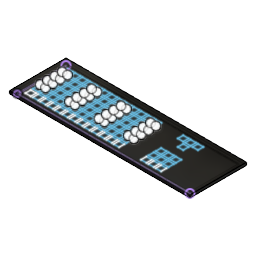
keyboard (Autodesk Fusion 360 design; units mm, degrees)
part number: 2026-07-05-21-32-07-139
Autodesk Fusion 360 part; units mm, degrees
sketch "Sketch1" plane through (0, 0, 0) normal (0, 1, 0) x (1, 0, 0)
  line L0 (0, 0) -> (446, 0)
  line L1 (446, 0) -> (446, -126)
  line L2 (446, -126) -> (0, -126)
  line L3 (0, -126) -> (0, 0)
  line L4 (-10, 10) -> (456, 10)
  line L5 (456, 10) -> (456, -136)
  line L6 (456, -136) -> (-10, -136)
  line L7 (-10, -136) -> (-10, 10)
  dimension "d1" = 446
  dimension "d2" = 126
  dimension "d3" = 466
  dimension "d4" = 146
  dimension "d5" = 10
  dimension "d6" = 10
  constraint horizontal L0
  constraint vertical L1
  constraint horizontal L2
  constraint vertical L3
  constraint coincident L0.start L3.end
  constraint horizontal L4
  constraint vertical L5
  constraint horizontal L6
  constraint vertical L7
  measures "d1" distance of L0.start L0.end
  measures "d2" distance of L0.start L2.end
  measures "d3" distance of L4.start L4.end
  measures "d4" distance of L4.start L6.end
  measures "d5" distance of L3 L7
  measures "d6" distance of L0 L4
extrude "Extrude1" add sketch "Sketch1" along normal blind 5 contours L0 L1 L2 L3 | L4 L5 L6 L7
extrude "Extrude2" cut sketch "Sketch1" along normal blind 4 contours L0 L1 L2 L3
extrude "Extrude3" add 1 faces at (145.3333, 5, 38.6667) along direction (0, 1, 0) blind 2
sketch "Sketch2" plane through (0, 0, 0) normal (0, 1, 0) x (1, 0, 0)
  line L0 (9, -114) -> (23, -114)
  line L1 (23, -114) -> (23, -100)
  line L2 (23, -100) -> (9, -100)
  line L3 (9, -100) -> (9, -114)
  line L4 (28, -113.6288) -> (42, -113.6288)
  line L5 (42, -113.6288) -> (42, -99.6288)
  line L6 (42, -99.6288) -> (28, -99.6288)
  line L7 (28, -99.6288) -> (28, -113.6288)
  line L8 (0, 0) -> (0, -126)
  line L9 (0, -126) -> (446, -126)
  line L10 (47, -113.6288) -> (61, -113.6288)
  line L11 (47, -99.6288) -> (47, -113.6288)
  line L12 (61, -113.6288) -> (61, -99.6288)
  line L13 (61, -99.6288) -> (47, -99.6288)
  line L14 (80, -113.6288) -> (80, -99.6288)
  line L15 (66, -113.6288) -> (80, -113.6288)
  line L16 (66, -99.6288) -> (66, -113.6288)
  line L17 (80, -99.6288) -> (66, -99.6288)
  line L18 (156, -113.6288) -> (156, -99.6288)
  line L19 (142, -113.6288) -> (156, -113.6288)
  line L20 (142, -99.6288) -> (142, -113.6288)
  line L21 (156, -99.6288) -> (142, -99.6288)
  line L22 (137, -113.6288) -> (137, -99.6288)
  line L23 (123, -99.6288) -> (123, -113.6288)
  line L24 (123, -113.6288) -> (137, -113.6288)
  line L25 (137, -99.6288) -> (123, -99.6288)
  line L26 (118, -113.6288) -> (118, -99.6288)
  line L27 (104, -113.6288) -> (118, -113.6288)
  line L28 (104, -99.6288) -> (104, -113.6288)
  line L29 (118, -99.6288) -> (104, -99.6288)
  line L30 (99, -114) -> (99, -100)
  line L31 (85, -114) -> (99, -114)
  line L32 (85, -100) -> (85, -114)
  line L33 (99, -100) -> (85, -100)
  line L34 (307.2, -113.6288) -> (321.2, -113.6288)
  line L35 (218, -113.6288) -> (232, -113.6288)
  line L36 (345.2, -113.6288) -> (359.2, -113.6288)
  line L37 (307.2, -99.6288) -> (307.2, -113.6288)
  line L38 (161, -114) -> (175, -114)
  line L39 (232, -113.6288) -> (232, -99.6288)
  line L40 (345.2, -99.6288) -> (345.2, -113.6288)
  line L41 (359.2, -99.6288) -> (345.2, -99.6288)
  line L42 (340.2, -113.6288) -> (340.2, -99.6288)
  line L43 (326.2, -99.6288) -> (326.2, -113.6288)
  line L44 (326.2, -113.6288) -> (340.2, -113.6288)
  line L45 (359.2, -113.6288) -> (359.2, -99.6288)
  line L46 (340.2, -99.6288) -> (326.2, -99.6288)
  line L47 (321.2, -113.6288) -> (321.2, -99.6288)
  line L48 (237, -114) -> (251, -114)
  line L49 (251, -114) -> (251, -100)
  line L50 (321.2, -99.6288) -> (307.2, -99.6288)
  line L51 (232, -99.6288) -> (218, -99.6288)
  line L52 (237, -100) -> (237, -114)
  line L53 (251, -100) -> (237, -100)
  line L54 (161, -100) -> (161, -114)
  line L55 (175, -114) -> (175, -100)
  line L56 (175, -100) -> (161, -100)
  line L57 (180, -99.6288) -> (180, -113.6288)
  line L58 (218, -99.6288) -> (218, -113.6288)
  line L59 (194, -113.6288) -> (194, -99.6288)
  line L60 (199, -113.6288) -> (213, -113.6288)
  line L61 (199, -99.6288) -> (199, -113.6288)
  line L62 (213, -113.6288) -> (213, -99.6288)
  line L63 (213, -99.6288) -> (199, -99.6288)
  line L64 (180, -113.6288) -> (194, -113.6288)
  line L65 (194, -99.6288) -> (180, -99.6288)
  line L66 (321.2, -94.6288) -> (321.2, -80.6288)
  line L67 (85, -95) -> (99, -95)
  line L68 (307.2, -80.6288) -> (307.2, -94.6288)
  line L69 (345.2, -94.6288) -> (359.2, -94.6288)
  line L70 (85, -81) -> (85, -95)
  line L71 (80, -80.6288) -> (66, -80.6288)
  line L72 (326.2, -94.6288) -> (340.2, -94.6288)
  line L73 (66, -94.6288) -> (80, -94.6288)
  line L74 (321.2, -80.6288) -> (307.2, -80.6288)
  line L75 (251, -95) -> (251, -81)
  line L76 (307.2, -94.6288) -> (321.2, -94.6288)
  line L77 (175, -81) -> (161, -81)
  line L78 (345.2, -80.6288) -> (345.2, -94.6288)
  line L79 (237, -81) -> (237, -95)
  line L80 (340.2, -94.6288) -> (340.2, -80.6288)
  line L81 (326.2, -80.6288) -> (326.2, -94.6288)
  line L82 (194, -80.6288) -> (180, -80.6288)
  line L83 (175, -95) -> (175, -81)
  line L84 (199, -80.6288) -> (199, -94.6288)
  line L85 (218, -94.6288) -> (232, -94.6288)
  line L86 (359.2, -80.6288) -> (345.2, -80.6288)
  line L87 (180, -80.6288) -> (180, -94.6288)
  line L88 (194, -94.6288) -> (194, -80.6288)
  line L89 (237, -95) -> (251, -95)
  line L90 (232, -94.6288) -> (232, -80.6288)
  line L91 (218, -80.6288) -> (218, -94.6288)
  line L92 (340.2, -80.6288) -> (326.2, -80.6288)
  line L93 (213, -80.6288) -> (199, -80.6288)
  line L94 (161, -95) -> (175, -95)
  line L95 (251, -81) -> (237, -81)
  line L96 (156, -94.6288) -> (156, -80.6288)
  line L97 (199, -94.6288) -> (213, -94.6288)
  line L98 (213, -94.6288) -> (213, -80.6288)
  line L99 (232, -80.6288) -> (218, -80.6288)
  line L100 (161, -81) -> (161, -95)
  line L101 (180, -94.6288) -> (194, -94.6288)
  line L102 (61, -94.6288) -> (61, -80.6288)
  line L103 (156, -80.6288) -> (142, -80.6288)
  line L104 (42, -80.6288) -> (28, -80.6288)
  line L105 (28, -80.6288) -> (28, -94.6288)
  line L106 (9, -81) -> (9, -95)
  line L107 (142, -94.6288) -> (156, -94.6288)
  line L108 (61, -80.6288) -> (47, -80.6288)
  line L109 (23, -81) -> (9, -81)
  line L110 (47, -94.6288) -> (61, -94.6288)
  line L111 (66, -80.6288) -> (66, -94.6288)
  line L112 (47, -80.6288) -> (47, -94.6288)
  line L113 (9, -95) -> (23, -95)
  line L114 (123, -80.6288) -> (123, -94.6288)
  line L115 (42, -94.6288) -> (42, -80.6288)
  line L116 (28, -94.6288) -> (42, -94.6288)
  line L117 (23, -95) -> (23, -81)
  line L118 (118, -94.6288) -> (118, -80.6288)
  line L119 (137, -80.6288) -> (123, -80.6288)
  line L120 (99, -81) -> (85, -81)
  line L121 (123, -94.6288) -> (137, -94.6288)
  line L122 (104, -94.6288) -> (118, -94.6288)
  line L123 (104, -80.6288) -> (104, -94.6288)
  line L124 (137, -94.6288) -> (137, -80.6288)
  line L125 (80, -94.6288) -> (80, -80.6288)
  line L126 (142, -80.6288) -> (142, -94.6288)
  line L127 (118, -80.6288) -> (104, -80.6288)
  line L128 (359.2, -94.6288) -> (359.2, -80.6288)
  line L129 (99, -95) -> (99, -81)
  line L130 (237, -62) -> (237, -76)
  line L131 (232, -61.6288) -> (218, -61.6288)
  line L132 (251, -62) -> (237, -62)
  line L133 (213, -75.6288) -> (213, -61.6288)
  line L134 (194, -75.6288) -> (194, -61.6288)
  line L135 (180, -61.6288) -> (180, -75.6288)
  line L136 (175, -62) -> (161, -62)
  line L137 (156, -75.6288) -> (156, -61.6288)
  line L138 (194, -61.6288) -> (180, -61.6288)
  line L139 (161, -62) -> (161, -76)
  line L140 (251, -76) -> (251, -62)
  line L141 (218, -61.6288) -> (218, -75.6288)
  line L142 (232, -75.6288) -> (232, -61.6288)
  line L143 (218, -75.6288) -> (232, -75.6288)
  line L144 (326.2, -61.6288) -> (326.2, -75.6288)
  line L145 (307.2, -61.6288) -> (307.2, -75.6288)
  line L146 (359.2, -75.6288) -> (359.2, -61.6288)
  line L147 (359.2, -61.6288) -> (345.2, -61.6288)
  line L148 (156, -61.6288) -> (142, -61.6288)
  line L149 (142, -75.6288) -> (156, -75.6288)
  line L150 (307.2, -75.6288) -> (321.2, -75.6288)
  line L151 (326.2, -75.6288) -> (340.2, -75.6288)
  line L152 (340.2, -61.6288) -> (326.2, -61.6288)
  line L153 (321.2, -61.6288) -> (307.2, -61.6288)
  line L154 (199, -75.6288) -> (213, -75.6288)
  line L155 (213, -61.6288) -> (199, -61.6288)
  line L156 (104, -75.6288) -> (118, -75.6288)
  line L157 (118, -75.6288) -> (118, -61.6288)
  line L158 (345.2, -75.6288) -> (359.2, -75.6288)
  line L159 (137, -75.6288) -> (137, -61.6288)
  line L160 (42, -75.6288) -> (42, -61.6288)
  line L161 (99, -76) -> (99, -62)
  line L162 (99, -62) -> (85, -62)
  line L163 (66, -61.6288) -> (66, -75.6288)
  line L164 (123, -61.6288) -> (123, -75.6288)
  line L165 (47, -75.6288) -> (61, -75.6288)
  line L166 (80, -75.6288) -> (80, -61.6288)
  line L167 (142, -61.6288) -> (142, -75.6288)
  line L168 (66, -75.6288) -> (80, -75.6288)
  line L169 (42, -61.6288) -> (28, -61.6288)
  line L170 (345.2, -61.6288) -> (345.2, -75.6288)
  line L171 (340.2, -75.6288) -> (340.2, -61.6288)
  line L172 (321.2, -75.6288) -> (321.2, -61.6288)
  line L173 (123, -75.6288) -> (137, -75.6288)
  line L174 (118, -61.6288) -> (104, -61.6288)
  line L175 (137, -61.6288) -> (123, -61.6288)
  line L176 (104, -61.6288) -> (104, -75.6288)
  line L177 (85, -62) -> (85, -76)
  line L178 (80, -61.6288) -> (66, -61.6288)
  line L179 (28, -75.6288) -> (42, -75.6288)
  line L180 (9, -62) -> (9, -76)
  line L181 (23, -62) -> (9, -62)
  line L182 (47, -61.6288) -> (47, -75.6288)
  line L183 (23, -76) -> (23, -62)
  line L184 (61, -61.6288) -> (47, -61.6288)
  line L185 (28, -61.6288) -> (28, -75.6288)
  line L186 (61, -75.6288) -> (61, -61.6288)
  line L187 (199, -61.6288) -> (199, -75.6288)
  line L188 (175, -76) -> (175, -62)
  line L189 (180, -75.6288) -> (194, -75.6288)
  line L190 (9, -76) -> (23, -76)
  line L191 (85, -76) -> (99, -76)
  line L192 (161, -76) -> (175, -76)
  line L193 (237, -76) -> (251, -76)
  line L194 (213, -42.6288) -> (199, -42.6288)
  line L195 (66, -56.6288) -> (80, -56.6288)
  line L196 (104, -56.6288) -> (118, -56.6288)
  line L197 (251, -43) -> (237, -43)
  line L198 (9, -43) -> (9, -57)
  line L199 (47, -42.6288) -> (47, -56.6288)
  line L200 (213, -56.6288) -> (213, -42.6288)
  line L201 (42, -42.6288) -> (28, -42.6288)
  line L202 (28, -42.6288) -> (28, -56.6288)
  line L203 (61, -56.6288) -> (61, -42.6288)
  line L204 (232, -56.6288) -> (232, -42.6288)
  line L205 (232, -42.6288) -> (218, -42.6288)
  line L206 (28, -56.6288) -> (42, -56.6288)
  line L207 (180, -42.6288) -> (180, -56.6288)
  line L208 (80, -42.6288) -> (66, -42.6288)
  line L209 (237, -43) -> (237, -57)
  line L210 (47, -56.6288) -> (61, -56.6288)
  line L211 (237, -57) -> (251, -57)
  line L212 (218, -42.6288) -> (218, -56.6288)
  line L213 (118, -42.6288) -> (104, -42.6288)
  line L214 (199, -56.6288) -> (213, -56.6288)
  line L215 (218, -56.6288) -> (232, -56.6288)
  line L216 (23, -57) -> (23, -43)
  line L217 (61, -42.6288) -> (47, -42.6288)
  line L218 (251, -57) -> (251, -43)
  line L219 (23, -43) -> (9, -43)
  line L220 (42, -56.6288) -> (42, -42.6288)
  line L221 (9, -57) -> (23, -57)
  line L222 (66, -42.6288) -> (66, -56.6288)
  line L223 (104, -42.6288) -> (104, -56.6288)
  line L224 (142, -56.6288) -> (156, -56.6288)
  line L225 (156, -42.6288) -> (142, -42.6288)
  line L226 (85, -57) -> (99, -57)
  line L227 (85, -43) -> (85, -57)
  line L228 (194, -56.6288) -> (194, -42.6288)
  line L229 (99, -57) -> (99, -43)
  line L230 (199, -42.6288) -> (199, -56.6288)
  line L231 (194, -42.6288) -> (180, -42.6288)
  line L232 (175, -43) -> (161, -43)
  line L233 (161, -43) -> (161, -57)
  line L234 (80, -56.6288) -> (80, -42.6288)
  line L235 (99, -43) -> (85, -43)
  line L236 (180, -56.6288) -> (194, -56.6288)
  line L237 (156, -56.6288) -> (156, -42.6288)
  line L238 (175, -57) -> (175, -43)
  line L239 (137, -56.6288) -> (137, -42.6288)
  line L240 (123, -56.6288) -> (137, -56.6288)
  line L241 (118, -56.6288) -> (118, -42.6288)
  line L242 (123, -42.6288) -> (123, -56.6288)
  line L243 (142, -42.6288) -> (142, -56.6288)
  line L244 (161, -57) -> (175, -57)
  line L245 (137, -42.6288) -> (123, -42.6288)
  line L246 (237, -5) -> (237, -19)
  line L247 (237, -38) -> (251, -38)
  line L248 (218, -37.6288) -> (232, -37.6288)
  line L249 (199, -37.6288) -> (213, -37.6288)
  line L250 (237, -24) -> (237, -38)
  line L251 (156, -4.6288) -> (142, -4.6288)
  line L252 (23, -19) -> (23, -5)
  line L253 (218, -18.6288) -> (232, -18.6288)
  line L254 (251, -24) -> (237, -24)
  line L255 (47, -4.6288) -> (47, -18.6288)
  line L256 (251, -5) -> (237, -5)
  line L257 (142, -18.6288) -> (156, -18.6288)
  line L258 (213, -37.6288) -> (213, -23.6288)
  line L259 (232, -23.6288) -> (218, -23.6288)
  line L260 (213, -18.6288) -> (213, -4.6288)
  line L261 (218, -4.6288) -> (218, -18.6288)
  line L262 (251, -19) -> (251, -5)
  line L263 (237, -19) -> (251, -19)
  line L264 (156, -23.6288) -> (142, -23.6288)
  line L265 (251, -38) -> (251, -24)
  line L266 (213, -4.6288) -> (199, -4.6288)
  line L267 (232, -4.6288) -> (218, -4.6288)
  line L268 (232, -18.6288) -> (232, -4.6288)
  line L269 (232, -37.6288) -> (232, -23.6288)
  line L270 (218, -23.6288) -> (218, -37.6288)
  line L271 (199, -18.6288) -> (213, -18.6288)
  line L272 (213, -23.6288) -> (199, -23.6288)
  line L273 (61, -18.6288) -> (61, -4.6288)
  line L274 (42, -18.6288) -> (42, -4.6288)
  line L275 (137, -18.6288) -> (137, -4.6288)
  line L276 (9, -5) -> (9, -19)
  line L277 (28, -4.6288) -> (28, -18.6288)
  line L278 (61, -4.6288) -> (47, -4.6288)
  line L279 (137, -4.6288) -> (123, -4.6288)
  line L280 (118, -18.6288) -> (118, -4.6288)
  line L281 (99, -19) -> (99, -5)
  line L282 (66, -37.6288) -> (80, -37.6288)
  line L283 (80, -23.6288) -> (66, -23.6288)
  line L284 (66, -18.6288) -> (80, -18.6288)
  line L285 (28, -18.6288) -> (42, -18.6288)
  line L286 (118, -23.6288) -> (104, -23.6288)
  line L287 (9, -19) -> (23, -19)
  line L288 (9, -24) -> (9, -38)
  line L289 (142, -4.6288) -> (142, -18.6288)
  line L290 (104, -4.6288) -> (104, -18.6288)
  line L291 (66, -4.6288) -> (66, -18.6288)
  line L292 (47, -23.6288) -> (47, -37.6288)
  line L293 (80, -18.6288) -> (80, -4.6288)
  line L294 (80, -4.6288) -> (66, -4.6288)
  line L295 (85, -5) -> (85, -19)
  line L296 (99, -5) -> (85, -5)
  line L297 (123, -4.6288) -> (123, -18.6288)
  line L298 (118, -4.6288) -> (104, -4.6288)
  line L299 (23, -5) -> (9, -5)
  line L300 (42, -4.6288) -> (28, -4.6288)
  line L301 (175, -38) -> (175, -24)
  line L302 (142, -37.6288) -> (156, -37.6288)
  line L303 (175, -24) -> (161, -24)
  line L304 (156, -37.6288) -> (156, -23.6288)
  line L305 (180, -23.6288) -> (180, -37.6288)
  line L306 (161, -19) -> (175, -19)
  line L307 (180, -18.6288) -> (194, -18.6288)
  line L308 (175, -5) -> (161, -5)
  line L309 (194, -4.6288) -> (180, -4.6288)
  line L310 (175, -19) -> (175, -5)
  line L311 (161, -24) -> (161, -38)
  line L312 (194, -37.6288) -> (194, -23.6288)
  line L313 (194, -23.6288) -> (180, -23.6288)
  line L314 (199, -23.6288) -> (199, -37.6288)
  line L315 (194, -18.6288) -> (194, -4.6288)
  line L316 (161, -5) -> (161, -19)
  line L317 (180, -4.6288) -> (180, -18.6288)
  line L318 (199, -4.6288) -> (199, -18.6288)
  line L319 (156, -18.6288) -> (156, -4.6288)
  line L320 (180, -37.6288) -> (194, -37.6288)
  line L321 (161, -38) -> (175, -38)
  line L322 (66, -23.6288) -> (66, -37.6288)
  line L323 (104, -23.6288) -> (104, -37.6288)
  line L324 (9, -38) -> (23, -38)
  line L325 (137, -23.6288) -> (123, -23.6288)
  line L326 (23, -38) -> (23, -24)
  line L327 (85, -24) -> (85, -38)
  line L328 (42, -37.6288) -> (42, -23.6288)
  line L329 (23, -24) -> (9, -24)
  line L330 (104, -37.6288) -> (118, -37.6288)
  line L331 (118, -37.6288) -> (118, -23.6288)
  line L332 (47, -18.6288) -> (61, -18.6288)
  line L333 (123, -18.6288) -> (137, -18.6288)
  line L334 (28, -23.6288) -> (28, -37.6288)
  line L335 (142, -23.6288) -> (142, -37.6288)
  line L336 (104, -18.6288) -> (118, -18.6288)
  line L337 (123, -23.6288) -> (123, -37.6288)
  line L338 (99, -38) -> (99, -24)
  line L339 (123, -37.6288) -> (137, -37.6288)
  line L340 (61, -37.6288) -> (61, -23.6288)
  line L341 (61, -23.6288) -> (47, -23.6288)
  line L342 (80, -37.6288) -> (80, -23.6288)
  line L343 (85, -38) -> (99, -38)
  line L344 (28, -37.6288) -> (42, -37.6288)
  line L345 (42, -23.6288) -> (28, -23.6288)
  line L346 (47, -37.6288) -> (61, -37.6288)
  line L347 (137, -37.6288) -> (137, -23.6288)
  line L348 (99, -24) -> (85, -24)
  line L349 (85, -19) -> (99, -19)
  line L350 (340.2, -37.6288) -> (340.2, -23.6288)
  line L351 (326.2, -23.6288) -> (326.2, -37.6288)
  line L352 (340.2, -23.6288) -> (326.2, -23.6288)
  line L353 (326.2, -37.6288) -> (340.2, -37.6288)
  line L354 (326.2, -18.6288) -> (340.2, -18.6288)
  line L355 (359.2, -4.6288) -> (345.2, -4.6288)
  line L356 (321.2, -4.6288) -> (307.2, -4.6288)
  line L357 (326.2, -4.6288) -> (326.2, -18.6288)
  line L358 (340.2, -18.6288) -> (340.2, -4.6288)
  line L359 (307.2, -18.6288) -> (321.2, -18.6288)
  line L360 (307.2, -4.6288) -> (307.2, -18.6288)
  line L361 (340.2, -4.6288) -> (326.2, -4.6288)
  line L362 (345.2, -18.6288) -> (359.2, -18.6288)
  line L363 (359.2, -18.6288) -> (359.2, -4.6288)
  line L364 (345.2, -4.6288) -> (345.2, -18.6288)
  line L365 (321.2, -18.6288) -> (321.2, -4.6288)
  dimension "d13" = 14
  dimension "d14" = 14
  dimension "d15" = 14
  dimension "d16" = 14
  dimension "d17" = 5
  dimension "d18" = 9
  dimension "d19" = 12
  dimension "d20" = 14
  dimension "d21" = 14
  dimension "d22" = 14
  dimension "d23" = 14
  dimension "d24" = 5
  dimension "d25" = 5
  dimension "d26" = 14
  dimension "d27" = 14
  dimension "d28" = 14
  dimension "d29" = 14
  dimension "d30" = 5
  dimension "d31" = 14
  dimension "d32" = 14
  dimension "d33" = 14
  dimension "d34" = 14
  dimension "d35" = 5
  dimension "d36" = 5
  dimension "d37" = 5
  dimension "d38" = 14
  dimension "d39" = 14
  dimension "d40" = 14
  dimension "d41" = 14
  dimension "d42" = 5
  dimension "d43" = 14
  dimension "d44" = 14
  dimension "d45" = 14
  dimension "d46" = 14
  dimension "d47" = 5
  dimension "d48" = 5
  dimension "d49" = 14
  dimension "d50" = 14
  dimension "d51" = 14
  dimension "d52" = 14
  dimension "d53" = 56.2
  dimension "d54" = 14
  dimension "d55" = 14
  dimension "d56" = 14
  dimension "d57" = 14
  dimension "d58" = 5
  dimension "d59" = 5
  dimension "d60" = 5
  dimension "d61" = 5
  dimension "d62" = 14
  dimension "d63" = 14
  dimension "d64" = 14
  dimension "d65" = 14
  dimension "d66" = 5
  dimension "d67" = 14
  dimension "d68" = 14
  dimension "d69" = 14
  dimension "d70" = 14
  dimension "d71" = 5
  dimension "d72" = 5
  dimension "d73" = 14
  dimension "d74" = 14
  dimension "d75" = 14
  dimension "d76" = 14
  dimension "d77" = 5
  dimension "d78" = 14
  dimension "d79" = 14
  dimension "d80" = 14
  dimension "d81" = 14
  dimension "d82" = 5
  dimension "d83" = 5
  dimension "d84" = 5
  dimension "d85" = 14
  dimension "d86" = 14
  dimension "d87" = 14
  dimension "d88" = 14
  dimension "d89" = 5
  dimension "d90" = 14
  dimension "d91" = 14
  dimension "d92" = 14
  dimension "d93" = 14
  dimension "d94" = 5
  dimension "d95" = 5
  dimension "d96" = 14
  dimension "d97" = 14
  dimension "d98" = 14
  dimension "d99" = 14
  dimension "d100" = 56.2
  dimension "d101" = 14
  dimension "d102" = 14
  dimension "d103" = 14
  dimension "d104" = 14
  dimension "d105" = 5
  dimension "d106" = 5
  dimension "d107" = 5
  dimension "d108" = 5
  dimension "d109" = 14
  dimension "d110" = 14
  dimension "d111" = 14
  dimension "d112" = 14
  dimension "d113" = 5
  dimension "d114" = 14
  dimension "d115" = 14
  dimension "d116" = 14
  dimension "d117" = 14
  dimension "d118" = 5
  dimension "d119" = 5
  dimension "d120" = 14
  dimension "d121" = 14
  dimension "d122" = 14
  dimension "d123" = 14
  dimension "d124" = 5
  dimension "d125" = 14
  dimension "d126" = 14
  dimension "d127" = 14
  dimension "d128" = 14
  dimension "d129" = 5
  dimension "d130" = 5
  dimension "d131" = 5
  dimension "d132" = 14
  dimension "d133" = 14
  dimension "d134" = 14
  dimension "d135" = 14
  dimension "d136" = 5
  dimension "d137" = 14
  dimension "d138" = 14
  dimension "d139" = 14
  dimension "d140" = 14
  dimension "d141" = 5
  dimension "d142" = 5
  dimension "d143" = 14
  dimension "d144" = 14
  dimension "d145" = 14
  dimension "d146" = 14
  dimension "d147" = 56.2
  dimension "d148" = 14
  dimension "d149" = 14
  dimension "d150" = 14
  dimension "d151" = 14
  dimension "d152" = 5
  dimension "d153" = 5
  dimension "d154" = 5
  dimension "d155" = 5
  dimension "d156" = 14
  dimension "d157" = 14
  dimension "d158" = 14
  dimension "d159" = 14
  dimension "d160" = 14
  dimension "d161" = 14
  dimension "d162" = 14
  dimension "d163" = 14
  dimension "d164" = 5
  dimension "d165" = 14
  dimension "d166" = 14
  dimension "d167" = 14
  dimension "d168" = 14
  dimension "d169" = 5
  dimension "d170" = 5
  dimension "d171" = 14
  dimension "d172" = 14
  dimension "d173" = 14
  dimension "d174" = 14
  dimension "d175" = 5
  dimension "d176" = 14
  dimension "d177" = 14
  dimension "d178" = 14
  dimension "d179" = 14
  dimension "d180" = 5
  dimension "d181" = 5
  dimension "d182" = 5
  dimension "d183" = 14
  dimension "d184" = 14
  dimension "d185" = 14
  dimension "d186" = 14
  dimension "d187" = 5
  dimension "d188" = 14
  dimension "d189" = 14
  dimension "d190" = 14
  dimension "d191" = 14
  dimension "d192" = 5
  dimension "d193" = 5
  dimension "d194" = 14
  dimension "d195" = 14
  dimension "d196" = 5
  dimension "d197" = 5
  dimension "d198" = 14
  dimension "d199" = 14
  dimension "d200" = 14
  dimension "d201" = 14
  dimension "d202" = 14
  dimension "d203" = 14
  dimension "d204" = 14
  dimension "d205" = 14
  dimension "d206" = 5
  dimension "d207" = 14
  dimension "d208" = 14
  dimension "d209" = 14
  dimension "d210" = 14
  dimension "d211" = 5
  dimension "d212" = 5
  dimension "d213" = 14
  dimension "d214" = 14
  dimension "d215" = 14
  dimension "d216" = 14
  dimension "d217" = 5
  dimension "d218" = 14
  dimension "d219" = 14
  dimension "d220" = 14
  dimension "d221" = 14
  dimension "d222" = 5
  dimension "d223" = 5
  dimension "d224" = 5
  dimension "d225" = 14
  dimension "d226" = 14
  dimension "d227" = 14
  dimension "d228" = 14
  dimension "d229" = 5
  dimension "d230" = 14
  dimension "d231" = 14
  dimension "d232" = 14
  dimension "d233" = 14
  dimension "d234" = 5
  dimension "d235" = 5
  dimension "d236" = 14
  dimension "d237" = 14
  dimension "d238" = 5
  dimension "d239" = 5
  dimension "d240" = 14
  dimension "d241" = 14
  dimension "d242" = 14
  dimension "d243" = 14
  dimension "d244" = 14
  dimension "d245" = 14
  dimension "d246" = 14
  dimension "d247" = 14
  dimension "d248" = 5
  dimension "d249" = 14
  dimension "d250" = 14
  dimension "d251" = 14
  dimension "d252" = 14
  dimension "d253" = 5
  dimension "d254" = 5
  dimension "d255" = 14
  dimension "d256" = 14
  dimension "d257" = 14
  dimension "d258" = 14
  dimension "d259" = 5
  dimension "d260" = 14
  dimension "d261" = 14
  dimension "d262" = 14
  dimension "d263" = 14
  dimension "d264" = 5
  dimension "d265" = 5
  dimension "d266" = 5
  dimension "d267" = 14
  dimension "d268" = 14
  dimension "d269" = 14
  dimension "d270" = 14
  dimension "d271" = 5
  dimension "d272" = 14
  dimension "d273" = 14
  dimension "d274" = 14
  dimension "d275" = 14
  dimension "d276" = 5
  dimension "d277" = 5
  dimension "d278" = 14
  dimension "d279" = 14
  dimension "d280" = 5
  dimension "d281" = 5
  dimension "d282" = 14
  dimension "d283" = 14
  dimension "d284" = 14
  dimension "d285" = 14
  dimension "d286" = 14
  dimension "d287" = 14
  dimension "d288" = 24
  dimension "d289" = 14
  dimension "d290" = 14
  dimension "d291" = 14
  dimension "d292" = 14
  dimension "d293" = 14
  dimension "d294" = 14
  dimension "d295" = 5
  dimension "d296" = 5
  constraint horizontal L0
  constraint vertical L1
  constraint horizontal L2
  constraint vertical L3
  constraint horizontal L4
  constraint vertical L5
  constraint horizontal L6
  constraint vertical L7
  constraint horizontal L10
  constraint vertical L12
  constraint horizontal L13
  constraint vertical L11
  constraint horizontal L15
  constraint vertical L14
  constraint horizontal L17
  constraint vertical L16
  constraint horizontal L31
  constraint vertical L30
  constraint horizontal L33
  constraint vertical L32
  constraint horizontal L27
  constraint vertical L26
  constraint horizontal L29
  constraint vertical L28
  constraint horizontal L24
  constraint vertical L22
  constraint horizontal L25
  constraint vertical L23
  constraint horizontal L19
  constraint vertical L18
  constraint horizontal L21
  constraint vertical L20
  constraint horizontal L38
  constraint vertical L55
  constraint horizontal L56
  constraint vertical L54
  constraint horizontal L64
  constraint vertical L59
  constraint horizontal L65
  constraint vertical L57
  constraint horizontal L60
  constraint vertical L62
  constraint horizontal L63
  constraint vertical L61
  constraint horizontal L35
  constraint vertical L39
  constraint horizontal L51
  constraint vertical L58
  constraint horizontal L48
  constraint vertical L49
  constraint horizontal L53
  constraint vertical L52
  constraint horizontal L34
  constraint vertical L47
  constraint horizontal L50
  constraint vertical L37
  constraint horizontal L44
  constraint vertical L42
  constraint horizontal L46
  constraint vertical L43
  constraint horizontal L36
  constraint vertical L45
  constraint horizontal L41
  constraint vertical L40
  constraint horizontal L113
  constraint vertical L117
  constraint horizontal L109
  constraint vertical L106
  constraint horizontal L116
  constraint vertical L115
  constraint horizontal L104
  constraint vertical L105
  constraint horizontal L110
  constraint vertical L102
  constraint horizontal L108
  constraint vertical L112
  constraint horizontal L73
  constraint vertical L125
  constraint horizontal L71
  constraint vertical L111
  constraint horizontal L67
  constraint vertical L129
  constraint horizontal L120
  constraint vertical L70
  constraint horizontal L122
  constraint vertical L118
  constraint horizontal L127
  constraint vertical L123
  constraint horizontal L121
  constraint vertical L124
  constraint horizontal L119
  constraint vertical L114
  constraint horizontal L107
  constraint vertical L96
  constraint horizontal L103
  constraint vertical L126
  constraint horizontal L94
  constraint vertical L83
  constraint horizontal L77
  constraint vertical L100
  constraint horizontal L101
  constraint vertical L88
  constraint horizontal L82
  constraint vertical L87
  constraint horizontal L97
  constraint vertical L98
  constraint horizontal L93
  constraint vertical L84
  constraint horizontal L85
  constraint vertical L90
  constraint horizontal L99
  constraint vertical L91
  constraint horizontal L89
  constraint vertical L75
  constraint horizontal L95
  constraint vertical L79
  constraint horizontal L76
  constraint vertical L66
  constraint horizontal L74
  constraint vertical L68
  constraint horizontal L72
  constraint vertical L80
  constraint horizontal L92
  constraint vertical L81
  constraint horizontal L69
  constraint vertical L128
  constraint horizontal L86
  constraint vertical L78
  constraint vertical L183
  constraint horizontal L181
  constraint vertical L180
  constraint horizontal L179
  constraint vertical L160
  constraint horizontal L169
  constraint vertical L185
  constraint horizontal L165
  constraint vertical L186
  constraint horizontal L184
  constraint vertical L182
  constraint horizontal L168
  constraint vertical L166
  constraint horizontal L178
  constraint vertical L163
  constraint vertical L161
  constraint horizontal L162
  constraint vertical L177
  constraint horizontal L156
  constraint vertical L157
  constraint horizontal L174
  constraint vertical L176
  constraint horizontal L173
  constraint vertical L159
  constraint horizontal L175
  constraint vertical L164
  constraint horizontal L149
  constraint vertical L137
  constraint horizontal L148
  constraint vertical L167
  constraint vertical L188
  constraint horizontal L136
  constraint vertical L139
  constraint horizontal L189
  constraint vertical L134
  constraint horizontal L138
  constraint vertical L135
  constraint horizontal L154
  constraint vertical L133
  constraint horizontal L155
  constraint vertical L187
  constraint horizontal L143
  constraint vertical L142
  constraint horizontal L131
  constraint vertical L141
  constraint vertical L140
  constraint horizontal L132
  constraint vertical L130
  constraint horizontal L150
  constraint vertical L172
  constraint horizontal L153
  constraint vertical L145
  constraint horizontal L151
  constraint vertical L171
  constraint horizontal L152
  constraint vertical L144
  constraint horizontal L158
  constraint vertical L146
  constraint horizontal L147
  constraint vertical L170
  constraint horizontal L190
  constraint horizontal L191
  constraint horizontal L192
  constraint horizontal L193
  constraint vertical L216
  constraint horizontal L219
  constraint vertical L198
  constraint horizontal L206
  constraint vertical L220
  constraint horizontal L201
  constraint vertical L202
  constraint horizontal L210
  constraint vertical L203
  constraint horizontal L217
  constraint vertical L199
  constraint horizontal L195
  constraint vertical L234
  constraint horizontal L208
  constraint vertical L222
  constraint vertical L229
  constraint horizontal L235
  constraint vertical L227
  constraint horizontal L196
  constraint vertical L241
  constraint horizontal L213
  constraint vertical L223
  constraint horizontal L240
  constraint vertical L239
  constraint horizontal L245
  constraint vertical L242
  constraint horizontal L224
  constraint vertical L237
  constraint horizontal L225
  constraint vertical L243
  constraint vertical L238
  constraint horizontal L232
  constraint vertical L233
  constraint horizontal L236
  constraint vertical L228
  constraint horizontal L231
  constraint vertical L207
  constraint horizontal L214
  constraint vertical L200
  constraint horizontal L194
  constraint vertical L230
  constraint horizontal L215
  constraint vertical L204
  constraint horizontal L205
  constraint vertical L212
  constraint vertical L218
  constraint horizontal L197
  constraint vertical L209
  constraint horizontal L221
  constraint horizontal L226
  constraint horizontal L244
  constraint horizontal L211
  constraint vertical L326
  constraint horizontal L329
  constraint vertical L288
  constraint horizontal L344
  constraint vertical L328
  constraint horizontal L345
  constraint vertical L334
  constraint horizontal L346
  constraint vertical L340
  constraint horizontal L341
  constraint vertical L292
  constraint horizontal L282
  constraint vertical L342
  constraint horizontal L283
  constraint vertical L322
  constraint vertical L338
  constraint horizontal L348
  constraint vertical L327
  constraint horizontal L330
  constraint vertical L331
  constraint horizontal L286
  constraint vertical L323
  constraint horizontal L339
  constraint vertical L347
  constraint horizontal L325
  constraint vertical L337
  constraint horizontal L302
  constraint vertical L304
  constraint horizontal L264
  constraint vertical L335
  constraint vertical L301
  constraint horizontal L303
  constraint vertical L311
  constraint horizontal L320
  constraint vertical L312
  constraint horizontal L313
  constraint vertical L305
  constraint horizontal L249
  constraint vertical L258
  constraint horizontal L272
  constraint vertical L314
  constraint horizontal L248
  constraint vertical L269
  constraint horizontal L259
  constraint vertical L270
  constraint vertical L265
  constraint horizontal L254
  constraint vertical L250
  constraint horizontal L324
  constraint horizontal L343
  constraint horizontal L321
  constraint horizontal L247
  constraint vertical L252
  constraint horizontal L299
  constraint vertical L276
  constraint horizontal L285
  constraint vertical L274
  constraint horizontal L300
  constraint vertical L277
  constraint horizontal L332
  constraint vertical L273
  constraint horizontal L278
  constraint vertical L255
  constraint horizontal L284
  constraint vertical L293
  constraint horizontal L294
  constraint vertical L291
  constraint vertical L281
  constraint horizontal L296
  constraint vertical L295
  constraint horizontal L336
  constraint vertical L280
  constraint horizontal L298
  constraint vertical L290
  constraint horizontal L333
  constraint vertical L275
  constraint horizontal L279
  constraint vertical L297
  constraint horizontal L257
  constraint vertical L319
  constraint horizontal L251
  constraint vertical L289
  constraint vertical L310
  constraint horizontal L308
  constraint vertical L316
  constraint horizontal L307
  constraint vertical L315
  constraint horizontal L309
  constraint vertical L317
  constraint horizontal L271
  constraint vertical L260
  constraint horizontal L266
  constraint vertical L318
  constraint horizontal L253
  constraint vertical L268
  constraint horizontal L267
  constraint vertical L261
  constraint vertical L262
  constraint horizontal L256
  constraint vertical L246
  constraint horizontal L287
  constraint horizontal L349
  constraint horizontal L306
  constraint horizontal L263
  constraint horizontal L353
  constraint vertical L350
  constraint horizontal L352
  constraint vertical L351
  constraint horizontal L359
  constraint vertical L365
  constraint horizontal L356
  constraint vertical L360
  constraint horizontal L354
  constraint vertical L358
  constraint horizontal L361
  constraint vertical L357
  constraint horizontal L362
  constraint vertical L363
  constraint horizontal L355
  constraint vertical L364
  measures "d13" distance of L0.start L0.end
  measures "d14" distance of L0.start L2.end
  measures "d15" distance of L4.start L4.end
  measures "d16" distance of L4.start L6.end
  measures "d17" distance of L1 L7
  measures "d18" distance of L3 L8
  measures "d19" distance of L0 L9
  measures "d20" distance of L10.end L10.start
  measures "d21" distance of L10.start L11.start
  measures "d22" distance of L14.start L15.start
  measures "d23" distance of L15.start L16.start
  measures "d24" distance of L5 L11
  measures "d25" distance of L12 L16
  measures "d26" distance of L31.start L30.start
  measures "d27" distance of L31.start L32.start
  measures "d28" distance of L26.start L27.start
  measures "d29" distance of L27.start L28.start
  measures "d30" distance of L28 L30
  measures "d31" distance of L22.start L23.end
  measures "d32" distance of L23.end L23.start
  measures "d33" distance of L18.start L19.start
  measures "d34" distance of L20.start L19.start
  measures "d35" distance of L23 L26
  measures "d36" distance of L20 L22
  measures "d37" distance of L14 L32
  measures "d38" distance of L38.start L38.end
  measures "d39" distance of L38.start L54.start
  measures "d40" distance of L59.start L57.end
  measures "d41" distance of L57.end L57.start
  measures "d42" distance of L55 L57
  measures "d43" distance of L60.end L60.start
  measures "d44" distance of L60.start L61.start
  measures "d45" distance of L35.end L35.start
  measures "d46" distance of L51.end L35.start
  measures "d47" distance of L59 L61
  measures "d48" distance of L58 L62
  measures "d49" distance of L48.end L48.start
  measures "d50" distance of L52.start L48.start
  measures "d51" distance of L34.start L34.end
  measures "d52" distance of L34.start L37.start
  measures "d53" distance of L37 L49
  measures "d54" distance of L42.start L43.end
  measures "d55" distance of L43.start L43.end
  measures "d56" distance of L36.end L36.start
  measures "d57" distance of L40.start L36.start
  measures "d58" distance of L43 L47
  measures "d59" distance of L40 L42
  measures "d60" distance of L39 L52
  measures "d61" distance of L18 L54
  measures "d62" distance of L106.end L113.end
  measures "d63" distance of L106.end L106.start
  measures "d64" distance of L115.start L105.end
  measures "d65" distance of L105.end L104.end
  measures "d66" distance of L105 L117
  measures "d67" distance of L102.start L110.start
  measures "d68" distance of L110.start L108.end
  measures "d69" distance of L73.end L73.start
  measures "d70" distance of L73.start L71.end
  measures "d71" distance of L112 L115
  measures "d72" distance of L102 L111
  measures "d73" distance of L67.start L67.end
  measures "d74" distance of L70.start L67.start
  measures "d75" distance of L122.start L118.start
  measures "d76" distance of L123.start L122.start
  measures "d77" distance of L123 L129
  measures "d78" distance of L114.end L121.end
  measures "d79" distance of L114.end L114.start
  measures "d80" distance of L96.start L107.start
  measures "d81" distance of L103.end L107.start
  measures "d82" distance of L114 L118
  measures "d83" distance of L124 L126
  measures "d84" distance of L70 L125
  measures "d85" distance of L94.start L83.start
  measures "d86" distance of L94.start L77.end
  measures "d87" distance of L88.start L87.end
  measures "d88" distance of L87.end L82.end
  measures "d89" distance of L83 L87
  measures "d90" distance of L97.end L84.end
  measures "d91" distance of L84.end L84.start
  measures "d92" distance of L85.end L85.start
  measures "d93" distance of L85.start L91.start
  measures "d94" distance of L84 L88
  measures "d95" distance of L91 L98
  measures "d96" distance of L79.end L75.start
  measures "d97" distance of L79.end L79.start
  measures "d98" distance of L68.end L66.start
  measures "d99" distance of L68.end L68.start
  measures "d100" distance of L68 L75
  measures "d101" distance of L72.end L72.start
  measures "d102" distance of L81.start L72.start
  measures "d103" distance of L69.end L69.start
  measures "d104" distance of L69.start L78.start
  measures "d105" distance of L66 L81
  measures "d106" distance of L78 L80
  measures "d107" distance of L79 L90
  measures "d108" distance of L96 L100
  measures "d109" distance of L180.end L183.start
  measures "d110" distance of L180.end L180.start
  measures "d111" distance of L179.start L160.start
  measures "d112" distance of L179.start L169.end
  measures "d113" distance of L183 L185
  measures "d114" distance of L165.start L165.end
  measures "d115" distance of L165.start L182.start
  measures "d116" distance of L163.end L166.start
  measures "d117" distance of L163.end L163.start
  measures "d118" distance of L160 L182
  measures "d119" distance of L163 L186
  measures "d120" distance of L177.end L161.start
  measures "d121" distance of L177.end L162.end
  measures "d122" distance of L156.start L156.end
  measures "d123" distance of L174.end L156.start
  measures "d124" distance of L161 L176
  measures "d125" distance of L164.end L159.start
  measures "d126" distance of L164.end L164.start
  measures "d127" distance of L137.start L149.start
  measures "d128" distance of L148.end L149.start
  measures "d129" distance of L157 L164
  measures "d130" distance of L159 L167
  measures "d131" distance of L166 L177
  measures "d132" distance of L188.start L139.end
  measures "d133" distance of L136.end L139.end
  measures "d134" distance of L134.start L135.end
  measures "d135" distance of L135.start L135.end
  measures "d136" distance of L135 L188
  measures "d137" distance of L154.start L133.start
  measures "d138" distance of L155.end L154.start
  measures "d139" distance of L142.start L141.end
  measures "d140" distance of L141.end L131.end
  measures "d141" distance of L134 L187
  measures "d142" distance of L133 L141
  measures "d143" distance of L130.end L140.start
  measures "d144" distance of L130.end L130.start
  measures "d145" distance of L145.end L150.end
  measures "d146" distance of L145.end L145.start
  measures "d147" distance of L140 L145
  measures "d148" distance of L151.end L144.end
  measures "d149" distance of L144.start L144.end
  measures "d150" distance of L158.start L146.start
  measures "d151" distance of L158.start L147.end
  measures "d152" distance of L144 L172
  measures "d153" distance of L170 L171
  measures "d154" distance of L130 L142
  measures "d155" distance of L137 L139
  measures "d156" distance of L180.end L183.start
  measures "d157" distance of L177.end L161.start
  measures "d158" distance of L188.start L139.end
  measures "d159" distance of L130.end L140.start
  measures "d160" distance of L198.end L216.start
  measures "d161" distance of L198.end L198.start
  measures "d162" distance of L202.end L206.end
  measures "d163" distance of L202.end L201.end
  measures "d164" distance of L202 L216
  measures "d165" distance of L199.end L203.start
  measures "d166" distance of L199.end L199.start
  measures "d167" distance of L195.start L195.end
  measures "d168" distance of L195.start L208.end
  measures "d169" distance of L199 L220
  measures "d170" distance of L203 L222
  measures "d171" distance of L226.end L226.start
  measures "d172" distance of L226.start L227.start
  measures "d173" distance of L196.start L196.end
  measures "d174" distance of L213.end L196.start
  measures "d175" distance of L223 L229
  measures "d176" distance of L240.start L239.start
  measures "d177" distance of L240.start L242.start
  measures "d178" distance of L224.start L224.end
  measures "d179" distance of L224.start L225.end
  measures "d180" distance of L241 L242
  measures "d181" distance of L239 L243
  measures "d182" distance of L227 L234
  measures "d183" distance of L238.start L233.end
  measures "d184" distance of L232.end L233.end
  measures "d185" distance of L207.end L228.start
  measures "d186" distance of L207.start L207.end
  measures "d187" distance of L207 L238
  measures "d188" distance of L200.start L214.start
  measures "d189" distance of L194.end L214.start
  measures "d190" distance of L204.start L212.end
  measures "d191" distance of L212.end L205.end
  measures "d192" distance of L228 L230
  measures "d193" distance of L200 L212
  measures "d194" distance of L209.end L211.end
  measures "d195" distance of L209.end L197.end
  measures "d196" distance of L204 L209
  measures "d197" distance of L233 L237
  measures "d198" distance of L198.end L216.start
  measures "d199" distance of L226.end L226.start
  measures "d200" distance of L238.start L233.end
  measures "d201" distance of L211.end L209.end
  measures "d202" distance of L288.end L324.end
  measures "d203" distance of L288.end L288.start
  measures "d204" distance of L334.end L328.start
  measures "d205" distance of L334.end L334.start
  measures "d206" distance of L326 L334
  measures "d207" distance of L292.end L340.start
  measures "d208" distance of L292.end L292.start
  measures "d209" distance of L282.start L282.end
  measures "d210" distance of L282.start L283.end
  measures "d211" distance of L292 L328
  measures "d212" distance of L322 L340
  measures "d213" distance of L338.start L327.end
  measures "d214" distance of L327.end L327.start
  measures "d215" distance of L323.end L330.end
  measures "d216" distance of L286.end L323.end
  measures "d217" distance of L323 L338
  measures "d218" distance of L337.end L339.end
  measures "d219" distance of L337.end L325.end
  measures "d220" distance of L302.start L302.end
  measures "d221" distance of L302.start L264.end
  measures "d222" distance of L331 L337
  measures "d223" distance of L335 L347
  measures "d224" distance of L327 L342
  measures "d225" distance of L301.start L311.end
  measures "d226" distance of L303.end L311.end
  measures "d227" distance of L305.end L312.start
  measures "d228" distance of L305.start L305.end
  measures "d229" distance of L301 L305
  measures "d230" distance of L249.end L249.start
  measures "d231" distance of L272.end L249.start
  measures "d232" distance of L248.end L248.start
  measures "d233" distance of L248.start L259.end
  measures "d234" distance of L312 L314
  measures "d235" distance of L258 L270
  measures "d236" distance of L247.start L247.end
  measures "d237" distance of L247.start L250.start
  measures "d238" distance of L250 L269
  measures "d239" distance of L304 L311
  measures "d240" distance of L288.end L324.end
  measures "d241" distance of L338.start L327.end
  measures "d242" distance of L301.start L311.end
  measures "d243" distance of L247.end L247.start
  measures "d244" distance of L276.end L252.start
  measures "d245" distance of L276.start L276.end
  measures "d246" distance of L277.end L274.start
  measures "d247" distance of L277.end L277.start
  measures "d248" distance of L252 L277
  measures "d249" distance of L255.end L273.start
  measures "d250" distance of L255.start L255.end
  measures "d251" distance of L284.start L284.end
  measures "d252" distance of L284.start L291.start
  measures "d253" distance of L255 L274
  measures "d254" distance of L273 L291
  measures "d255" distance of L295.end L281.start
  measures "d256" distance of L295.end L295.start
  measures "d257" distance of L290.end L280.start
  measures "d258" distance of L290.start L290.end
  measures "d259" distance of L281 L290
  measures "d260" distance of L275.start L297.end
  measures "d261" distance of L297.end L279.end
  measures "d262" distance of L257.start L257.end
  measures "d263" distance of L257.start L251.end
  measures "d264" distance of L280 L297
  measures "d265" distance of L275 L289
  measures "d266" distance of L293 L295
  measures "d267" distance of L306.end L306.start
  measures "d268" distance of L308.end L306.start
  measures "d269" distance of L307.end L307.start
  measures "d270" distance of L309.end L307.start
  measures "d271" distance of L310 L317
  measures "d272" distance of L260.start L271.start
  measures "d273" distance of L266.end L271.start
  measures "d274" distance of L253.end L253.start
  measures "d275" distance of L261.start L253.start
  measures "d276" distance of L315 L318
  measures "d277" distance of L260 L261
  measures "d278" distance of L246.end L262.start
  measures "d279" distance of L246.end L246.start
  measures "d280" distance of L246 L268
  measures "d281" distance of L316 L319
  measures "d282" distance of L276.end L252.start
  measures "d283" distance of L281.start L295.end
  measures "d284" distance of L306.end L306.start
  measures "d285" distance of L262.start L246.end
  measures "d286" distance of L351.end L350.start
  measures "d287" distance of L351.start L351.end
  measures "d288" distance of L152 L353
  measures "d289" distance of L359.end L359.start
  measures "d290" distance of L356.end L359.start
  measures "d291" distance of L354.start L354.end
  measures "d292" distance of L357.start L354.start
  measures "d293" distance of L362.end L362.start
  measures "d294" distance of L355.end L362.start
  measures "d295" distance of L357 L365
  measures "d296" distance of L358 L364
